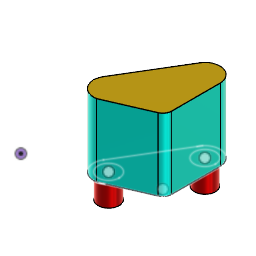
Fender (Autodesk Fusion 360 design; units mm, degrees)
part number: 2026-05-25-19-31-43-206
Autodesk Fusion 360 part; units mm, degrees
sketch "Sketch1" plane through (0, 0, 0) normal (0, 0, 1) x (1, 0, 0)
  line L0 (10.392, 2.2094) -> (17.5059, 5.2858)
  line L1 (13.949, 16.2125) -> (7.769, 5.9525)
  line L2 (18.4095, 14.7335) -> (18.4105, 6.6627)
  arc A0 (7.769, 5.9525) -> (11.3682, 2.6315) centre (9.9105, 4.6625) ccw
  circle A1 centre (9.9105, 4.6625) radius 1.75
  circle A2 centre (15.9105, 14.6625) radius 1.75
  arc A3 (17.5059, 5.2858) -> (18.4105, 6.6627) centre (16.9105, 6.6625) ccw
  arc A4 (18.4095, 14.5922) -> (13.6233, 15.6718) centre (15.9105, 14.6625) ccw
  dimension "d1" = 5
  dimension "d2" = 5
  dimension "d3" = 3
  dimension "d4" = 3.5
  dimension "d5" = 3.5
  dimension "d6" = 9.9105
  dimension "d7" = 4.6625
  dimension "d8" = 7.1139
  dimension "d9" = 3.0764
  dimension "d10" = 11.3682
  dimension "d11" = 8.0707
  dimension "d12" = 5.9525
  dimension "d13" = 16.2125
  dimension "d14" = 6.6627
  constraint coincident L0.start A0
  constraint tangent L0 A3
  constraint coincident L2.start A4
  constraint tangent L2 A3
  constraint coincident L1.start A4
  constraint tangent L1 A0
  constraint coincident A4.end L1
  constraint coincident A4.start L2
  constraint coincident A0.end L0
  constraint concentric A0 A1
  constraint concentric A2 A4
  measures "d1" diameter of A0
  measures "d2" diameter of A4
  measures "d3" diameter of A3
  measures "d4" diameter of A1
  measures "d5" diameter of A2
  measures "d6" horizontal distance of origin A0.centre
  measures "d7" vertical distance of origin A0.centre
  measures "d8" horizontal distance of L0.end L0.start
  measures "d9" vertical distance of L0.end L0.start
  measures "d10" horizontal distance of origin A0.end
  measures "d11" vertical distance of L2.end L2.start
  measures "d12" vertical distance of origin L1.end
  measures "d13" vertical distance of origin L1.start
  measures "d14" vertical distance of origin L2.end
extrude "Extrude1" add sketch "Sketch1" along normal blind 12 contours L0 L1 L2 A0 A3 A4
extrude "Extrude2" add sketch "Sketch1" along normal blind 16 from surface at -4 contours A1 | A2
